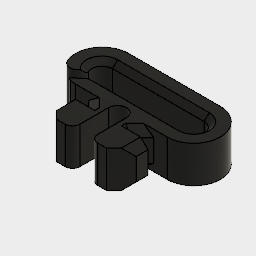
cable_clip_lcd (Autodesk Fusion 360 design; units mm, degrees)
Autodesk Fusion 360 part; units mm, degrees
sketch "base" plane through (0, 0, 0) normal (0, 0, 1) x (1, 0, 0)
  line L0 (-3.4, 0) -> (-2.2, 0)
  arc A0 (-2.2, 0) -> (-1.2, 1) centre (-2.2, 1) ccw
  line L1 (-1.2, 1) -> (-1.2, 4.9)
  line L2 (-3.4, 0) -> (-5.4, 2)
  line L3 (-5.4, 3.6) -> (-2.8, 3.6)
  line L4 (-2.8, 3.8) -> (-4.4, 5.4)
  line L5 (-2.2, 0) -> (0, 0) construction
  line L6 (-5.4, 3.6) -> (-5.4, 2)
  line L7 (0, 7.6) -> (-6.2, 7.6)
  arc A1 (-6.2, 10.4) -> (-6.2, 7.6) centre (-6.2, 9) ccw
  line L8 (-6.2, 10.4) -> (0, 10.4)
  line L9 (-4.4, 5.4) -> (-6.2, 5.4)
  arc A2 (-6.2, 12.6) -> (-6.2, 5.4) centre (-6.2, 9) ccw
  line L10 (-6.2, 12.6) -> (0, 12.6)
  line L11 (0, 12.6) -> (0, 0) construction
  line L12 (-2.8, 3.8) -> (-2.8, 3.6)
  arc A3 (6.2, 7.6) -> (6.2, 10.4) centre (6.2, 9) ccw
  line L13 (6.2, 10.4) -> (0, 10.4)
  line L14 (0, 7.6) -> (6.2, 7.6)
  arc A4 (0, 6.1) -> (-1.2, 4.9) centre (0, 4.9) ccw
  line L15 (6.2, 12.6) -> (0, 12.6)
  arc A5 (6.2, 5.4) -> (6.2, 12.6) centre (6.2, 9) ccw
  line L16 (4.4, 5.4) -> (6.2, 5.4)
  line L17 (2.8, 3.8) -> (4.4, 5.4)
  line L18 (2.8, 3.8) -> (2.8, 3.6)
  line L19 (5.4, 3.6) -> (2.8, 3.6)
  line L20 (5.4, 3.6) -> (5.4, 2)
  line L21 (3.4, 0) -> (5.4, 2)
  line L22 (3.4, 0) -> (2.2, 0)
  arc A6 (1.2, 1) -> (2.2, 0) centre (2.2, 1) ccw
  arc A7 (1.2, 4.9) -> (0, 6.1) centre (0, 4.9) ccw
  line L23 (1.2, 1) -> (1.2, 4.9)
  line L24 (-6.2, 7.6) -> (-7.2689, 6.7031)
  arc A8 (-9.5116, 7.5881) -> (-7.4878, 8.4509) centre (-8.4997, 8.0195) ccw
  line L25 (-6.2, 9) -> (-9.5116, 7.5881) construction
  arc A9 (-7.2689, 6.7031) -> (-6.9684, 5.483) centre (-6.819, 6.1668) ccw
  dimension "d6" = 4.2
  dimension "d7" = 135
  dimension "d8" = 45
  dimension "d9" = 1
  dimension "d10" = 1.2
  dimension "d17" = 2.2
  dimension "d18" = 2.8
  dimension "d20" = 6.2
  dimension "d27" = 0.2
  dimension "d28" = 2.6
  dimension "d29" = 1.6
  dimension "d31" = 2
  dimension "d32" = 1.8
  dimension "d33" = 1.5
  dimension "d58" = 0.6996
  dimension "d59" = 0.7
  dimension "d60" = 140
  measures "d6" distance of A0.end L6
  measures "d7" angle of L0 L2
  measures "d8" angle of L3 L4
  measures "d9" radius of A0
  measures "d10" distance of L5.end L1
  measures "d17" distance of A1 A2
  measures "d18" distance of L7 L8
  measures "d20" distance of A1.centre L10.end
  measures "d27" distance of L4.start L3.end
  measures "d28" distance of L6 L3.end
  measures "d29" distance of L2.end L3.start
  measures "d31" distance of L0.start L2.end
  measures "d32" distance of L3.start L9
  measures "d33" distance of L7.start A4.start
  measures "d58" distance of L24 A8
  measures "d59" radius of A9
  measures "d60" angle of L7 L24
extrude "Extrude1" add sketch "base" along normal blind 5 contours L0 A0 L1 L2 L3 L4 L6 L7 A1 L8 L9 A2 L10 L12 A3 L13 L14 A4 L15 A5 L16 L17 L18 L19 L20 L21 L22 A6 A7 L23 L24 A8 A9
fillet "Fillet1" radius 0.8 1 edges at (-6.2, 7.6, 2.5)
chamfer "Chamfer1" distance 1 angle 45 12 edges at (-5.4, 2.8, 5) (-5.4, 2.8, 0) (5.4, 2.8, 0) (5.4, 2.8, 5) (-3.6, 4.6, 5) (-2.8, 3.7, 5) (2.8, 3.7, 5) (3.6, 4.6, 5) (2.8, 3.7, 0) (3.6, 4.6, 0) (-3.6, 4.6, 0) (-2.8, 3.7, 0)
chamfer "Chamfer3" distance 0.7 angle 45 12 edges at (0.1456, 7.6, 0) (7.6, 9, 0) (0, 10.4, 5) (7.6, 9, 5) (0, 10.4, 0) (-7.3681, 9.7718, 0) (0.1456, 7.6, 5) (-7.3681, 9.7718, 5) (-6.1824, 7.5518, 5) (-6.846, 7.0579, 5) (-6.1824, 7.5518, 0) (-6.846, 7.0579, 0) tangent chain off
